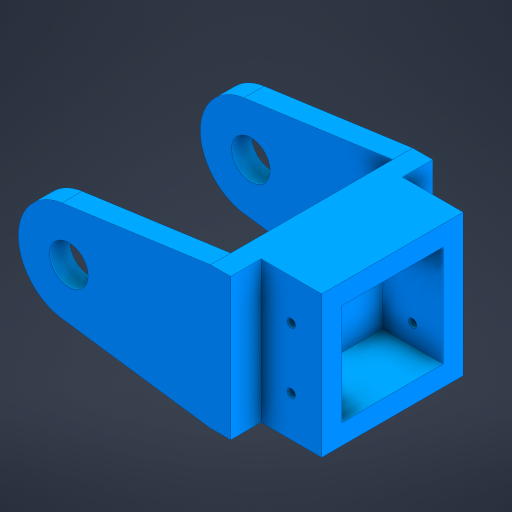
# Autodesk Inventor part: Forearm-End Fork
Saved by Autodesk Inventor 2023 (Build 270158000, 158)
## iProperties
Created: 2023-08-18
Part Number: Forearm-End Fork
Material: Acrylic, Clear
Document SubType Name: Modeling
Designer: Abhinav
Density: 1.19 g/cm^3
Appearance: Generic(1)
Mass: 285.375 g
Surface Area: 560.575 cm^2
Volume: 239.811 cm^3
Author: Abhinav
Autodesk Inventor part; units mm, degrees
ref_plane "YZ Plane" through (0, 0, 0) normal (1, 0, 0) x (0, 1, 0)
ref_plane "XZ Plane" through (0, 0, 0) normal (0, 1, 0) x (-1, 0, 0)
sketch "Sketch1" plane through (0, 0, 0) normal (0, 0, 1) x (1, 0, 0)
  circle A0 centre (0, 0) radius 9.5
  line L0 (70, 35) -> (80, 35)
  line L1 (80, 35) -> (80, -35)
  line L2 (80, -35) -> (70, -35)
  line L3 (70, -35) -> (70, 35)
  line L4 (70, 35) -> (80, -35) construction
  line L5 (80, 35) -> (70, -35) construction
  arc A1 (-3.4517, 24.7606) -> (-3.4517, -24.7606) centre (0, 0) ccw
  line L6 (70, 35) -> (-3.4517, 24.7606)
  line L7 (70, -35) -> (-3.4517, -24.7606)
  line L8 (0, 0) -> (70, 0)
  point P0 (75, 0)
  dimension "d0" = 19
  dimension "d11" = 10
  dimension "d12" = 70
  dimension "d13" = 50
  dimension "d25" = 70
  constraints: 18 end point, 3 midpoint, 2 centre point, 2 coincident, 2 parallel, 2 point on circle, 2 tangent, 1 horizontal, 1 perpendicular
  measures "d0" diameter of A0
  measures "d11" distance of L1.end L2.end
  measures "d12" distance of L0.end L1.end
  measures "d13" diameter of A1
  measures "d25" distance of L8.start L8.end
extrude "Extrusion1" add sketch "Sketch1" along normal blind 10
ref_plane "Work Plane1" through (0, 0, -80) normal (0, 0, -1) x (-1, 0, 0)
sketch "Sketch2" plane through (0, 0, -80) normal (0, 0, -1) x (-1, 0, 0)
  circle A0 centre (0, 0) radius 9.5 projected
  arc A1 (3.4517, -24.7606) -> (3.4517, 24.7606) centre (0, 0) ccw projected
  line L0 (-70, 35) -> (3.4517, 24.7606) projected
  line L1 (-80, 35) -> (-70, 35) projected
  line L2 (-80, -35) -> (-80, 35) projected
  line L3 (-70, -35) -> (-80, -35) projected
  line L4 (3.4517, -24.7606) -> (-70, -35) projected
  circle A2 centre (0, 0) radius 9.5 projected
extrude "Extrusion2" add sketch "Sketch2" along normal blind 10
extrude "Extrusion3" add sketch "Sketch1" against normal blind 80 contours L3 L0 L1 L2
sketch "Sketch3" plane through (80, -35, 10) normal (1, 0, 0) x (0, 0, -1)
  line L0 (0, 0) -> (0, 70) construction
  line L1 (0, 70) -> (100, 0) construction
  line L2 (100, 0) -> (0, 0) projected
  line L3 (15, 70) -> (85, 70)
  line L4 (85, 70) -> (85, 0)
  line L5 (85, 0) -> (15, 0)
  line L6 (15, 0) -> (15, 70)
  line L7 (15, 70) -> (85, 0) construction
  line L8 (85, 70) -> (15, 0) construction
  line L9 (25, 60) -> (75, 60)
  line L10 (75, 60) -> (75, 10)
  line L11 (75, 10) -> (25, 10)
  line L12 (25, 10) -> (25, 60)
  line L13 (25, 60) -> (75, 10) construction
  line L14 (75, 60) -> (25, 10) construction
  point P0 (10, 35)
  point P1 (50, 35)
  point P2 (50, 35)
  point P3 (15, 0)
  point P4 (160, 0)
  dimension "d14" = 70
  dimension "d15" = 50
  dimension "d16" = 50
  constraints: 26 end point, 6 midpoint, 4 parallel, 2 horizontal, 2 perpendicular, 1 point on line
  measures "d14" distance of L4.end L5.end
  measures "d15" distance of L10.end L11.end
  measures "d16" distance of L9.end L10.end
extrude "Extrusion4" add sketch "Sketch3" along normal blind 30
sketch "Sketch4" plane through (70, 35, -75) normal (0, 0, -1) x (1, 0, 0)
  line L0 (10, 0) -> (40, 0) construction
  line L1 (40, 70) -> (40, 0) construction
  line L2 (10, 0) -> (40, 70) construction
  line L3 (25, 35) -> (25, 50) construction
  line L4 (25, 50) -> (25, 20) construction
  circle A0 centre (25, 50) radius 2
  circle A1 centre (25, 20) radius 2
  point P0 (-70, 35)
  dimension "d19" = 15
  dimension "d20" = 30
  dimension "d21" = 4
  dimension "d22" = 4
  constraints: 6 end point, 2 centre point, 2 coincident, 1 midpoint, 1 point on line, 1 vertical
  measures "d19" distance of L3.start L3.end
  measures "d20" distance of L3.end L4.end
  measures "d21" diameter of A0
  measures "d22" diameter of A1
extrude "Extrusion5" cut sketch "Sketch4" against normal blind 70
body "Solid1"
